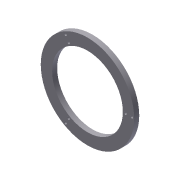
# Autodesk Inventor part: ring_top
Saved by Autodesk Inventor 2012 (Build 160160000, 160)
## iProperties
Created: 2012-04-25
Part Number: ring_top
Material: Aluminum-6061
Document SubType Name: Modeling
Designer: Antonella Wilby
Density: 2.71 g/cm^3
Mass: 488.302 g
Surface Area: 425.634 cm^2
Volume: 180.185 cm^3
Author: Antonella Wilby
Autodesk Inventor part; units mm, degrees
ref_plane "YZ Plane" through (0, 0, 0) normal (1, 0, 0) x (0, 1, 0)
ref_plane "XZ Plane" through (0, 0, 0) normal (0, 1, 0) x (-1, 0, 0)
ref_plane "XY Plane" through (0, 0, 0) normal (0, 0, 1) x (1, 0, 0)
sketch "Sketch1" plane through (0, 0, 0) normal (0, 0, 1) x (1, 0, 0)
  circle A0 centre (0, 0) radius 88.9
  circle A1 centre (0, 0) radius 117.475
  dimension "d0" = 177.8
  dimension "d2" = 28.575
  constraints: 2 centre point, 2 coincident
  measures "d0" diameter of A0
  measures "d2" radial gap between concentric circles of A1 A0
extrude "Extrusion1" add sketch "Sketch1" along normal mid plane 12.7
sketch "Sketch2" plane through (0, 0, 6.35) normal (0, 0, 1) x (1, 0, 0)
  circle A0 centre (0, 0) radius 117.475 projected
  line L0 (0, 0) -> (-47.625, 82.4889) construction
  line L1 (-164.465, 0) -> (164.465, 0) projected
  line L2 (0, -164.465) -> (0, 164.465) projected
  line L3 (-47.625, 82.4889) -> (-55.5625, 96.2371) construction
  dimension "d5" = 30
  dimension "d16" = 95.25
  dimension "d17" = 15.875
  constraints: 4 end point, 1 collinear
  measures "d5" angle of L2 L0
  measures "d16" distance of L0.start L0.end
  measures "d17" distance of L3.end L0.end
hole "Hole1" at (-47.625, 82.4889, 6.35) at (-55.5625, 96.2371, 6.35) direction (0, 0, -1) diameter 6.35 end through all
pattern_circular "Circular Pattern1" count 3 over 360 about axis through (0, 0, -10) along (0, 0, 1) of "Hole1"
body "Solid1"
